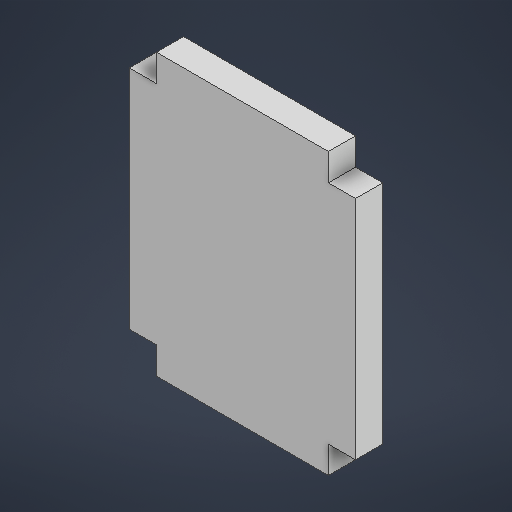
# Autodesk Inventor part: Frontrail
Saved by Autodesk Inventor 2027 (Build 310192000, 192)
## iProperties
Created: 2026-05-09
Part Number: Frontrail
Material: Generic
Document SubType Name: Modeling
Designer: alexy
Density: 1 g/cm^3
Appearance: Default
Author: alexy
Autodesk Inventor part; units mm, degrees
ref_plane "YZ Plane" through (0, 0, 0) normal (1, 0, 0) x (0, 1, 0)
ref_plane "XZ Plane" through (0, 0, 0) normal (0, 1, 0) x (-1, 0, 0)
ref_plane "XY Plane" through (0, 0, 0) normal (0, 0, 1) x (1, 0, 0)
sketch "Sketch1" plane through (0, 0, 0) normal (0, 0, 1) x (1, 0, 0)
  line L0 (0, 0) -> (19, 0)
  line L1 (19, 0) -> (19, 31)
  line L2 (19, 31) -> (0, 31)
  line L3 (0, 31) -> (0, 0)
  line L4 (-3, 28) -> (0, 28)
  line L5 (0, 28) -> (0, 3)
  line L6 (0, 3) -> (-3, 3)
  line L7 (-3, 3) -> (-3, 28)
  line L8 (-3, 28) -> (0, 3) construction
  line L9 (0, 28) -> (-3, 3) construction
  line L10 (22, 28) -> (19, 28)
  line L11 (19, 28) -> (19, 3)
  line L12 (19, 3) -> (22, 3)
  line L13 (22, 3) -> (22, 28)
  line L14 (22, 28) -> (19, 3) construction
  line L15 (19, 28) -> (22, 3) construction
  point P0 (-1.5, 15.5)
  point P1 (20.5, 15.5)
  point P2 (0, 15.5)
  point P3 (0, 15.5)
  point P4 (0, 28)
  dimension "d0" = 19
  dimension "d1" = 31
  dimension "d2" = 3
  dimension "d3" = 3
  dimension "d4" = 25
  constraints: 32 end point, 6 midpoint, 6 parallel, 3 horizontal, 3 perpendicular, 3 point on line, 2 horizontal alignment
  measures "d0" distance of L2.end L1.end
  measures "d1" distance of L0.end L1.end
  measures "d2" distance of L10.start L10.end
  measures "d3" distance of L4.start L4.end
  measures "d4" distance of L6.end L4.start
extrude "Extrusion1" add sketch "Sketch1" along normal blind 3
body "Solid1"
